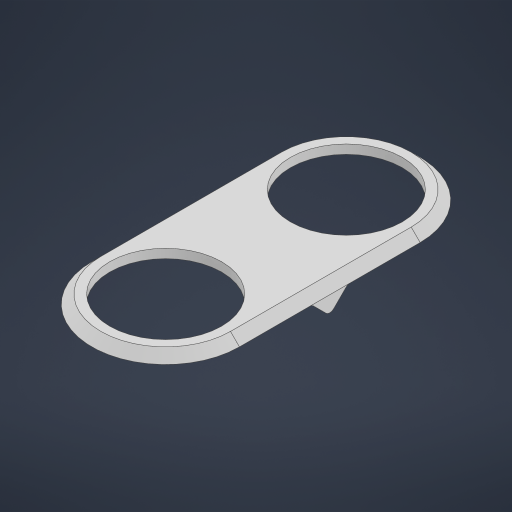
# Autodesk Inventor part: Ultrasonic Sensor Cover
Saved by Autodesk Inventor 2024 (Build 280153000, 153)
## iProperties
Created: 2026-03-21
Part Number: Ultrasonic Sensor Cover
Material: Generic
Document SubType Name: Modeling
Designer: Vincent Larson
Density: 1 g/cm^3
Appearance: Default
Author: Vincent Larson
Autodesk Inventor part; units mm, degrees
ref_plane "YZ Plane" through (0, 0, 0) normal (1, 0, 0) x (0, 1, 0)
ref_plane "XZ Plane" through (0, 0, 0) normal (0, 1, 0) x (-1, 0, 0)
ref_plane "XY Plane" through (0, 0, 0) normal (0, 0, 1) x (1, 0, 0)
sketch "Sketch1" plane through (0, 0, 0) normal (0, 1, 0) x (-1, 0, 0)
  circle A0 centre (0, 0) radius 7.9375
  line L0 (0, -7.9375) -> (0, -17.7165)
  line L1 (0, -17.7165) -> (0, -33.5915)
  circle A1 centre (0, -25.654) radius 7.9375
  line L2 (0, 0) -> (0, -25.654) construction
  line L3 (-7.9375, 0) -> (-7.9375, -25.654)
  line L4 (7.9375, -25.654) -> (7.9375, 0)
  arc A2 (7.9375, 0) -> (-7.9375, 0) centre (0, 0) ccw
  arc A3 (-7.9375, -25.654) -> (7.9375, -25.654) centre (0, -25.654) ccw
  line L5 (10.4775, 0) -> (10.4775, -25.654)
  arc A4 (-10.4775, -25.654) -> (10.4775, -25.654) centre (0, -25.654) ccw
  line L6 (-10.4775, -25.654) -> (-10.4775, 0)
  arc A5 (10.4775, 0) -> (-10.4775, 0) centre (0, 0) ccw
  point P0 (0, -12.827)
  dimension "d0" = 15.875
  dimension "d1" = 9.779
  dimension "d2" = 15.875
  dimension "d3" = 2.54
  constraints: 16 end point, 8 point on circle, 4 centre point, 4 tangent, 2 midpoint, 2 parallel, 2 vertical, 2 vertical alignment, 1 coincident, 1 collinear, 8 other
  measures "d1" distance of L0.start L0.end
  measures "d2" distance of L0.end L1.end
  measures "d3" distance between parallel lines of L4 L5
extrude "Extrusion1" add sketch "Sketch1" along normal blind 1.27 contours L4 A1 L0 A0 | A0 L0 A1 L3 | L5 A4 L6 A5
sketch "Sketch2" plane through (10.4775, 0, 0) normal (1, 0, 0) x (0, 0, -1)
  line L0 (25.654, 0) -> (0, 0) projected
  line L1 (12.827, 0) -> (12.827, -2.54)
  line L2 (12.827, -2.54) -> (10.287, 0)
  line L3 (12.827, -2.54) -> (15.367, 0)
  dimension "d6" = 2.54
  dimension "d7" = 45
  constraints: 6 end point, 2 point on line, 1 midpoint, 1 vertical
  measures "d6" distance of L1.start L1.end
  measures "d7" angle of L1 L2
extrude "Extrusion2" add sketch "Sketch2" against normal up to surface (20.955 mm away)
fillet "Fillet1" radius 0.762 3 edges at (0, 0, -15.367) (0, -2.54, -12.827) (0, 0, -10.287)
chamfer "Chamfer1" distance 1.27 angle 45 4 edges at (10.4775, 1.27, -12.827) (0, 1.27, -36.1315) (-10.4775, 1.27, -12.827) (0, 1.27, 10.4775)
body "Solid1"
